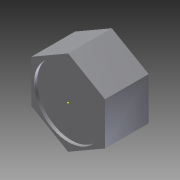
# Autodesk Inventor part: Поз10 Заглушка
Saved by Autodesk Inventor 2012 SP2 (Build 160219200, 219)
## iProperties
Created: 2014-04-06
Part Number: Поз10 Заглушка
Material: Default
Document SubType Name: Modeling
Designer: N750
Density: 1 g/cm^3
Author: N750
Autodesk Inventor part; units mm, degrees
ref_plane "YZ Plane" through (0, 0, 0) normal (1, 0, 0) x (0, 1, 0)
ref_plane "XZ Plane" through (0, 0, 0) normal (0, 1, 0) x (-1, 0, 0)
ref_plane "XY Plane" through (0, 0, 0) normal (0, 0, 1) x (1, 0, 0)
sketch "Эскиз1" plane through (0, 0, 0) normal (0, 0, 1) x (1, 0, 0)
  point P0 (0, 0)
sketch "Эскиз2" plane through (0, 0, 0) normal (0, 1, 0) x (-1, 0, 0)
  line L0 (0, 15.5885) -> (13.5, 7.7942)
  line L1 (13.5, 7.7942) -> (13.5, -7.7942)
  line L2 (13.5, -7.7942) -> (0, -15.5885)
  line L3 (0, -15.5885) -> (-13.5, -7.7942)
  line L4 (-13.5, -7.7942) -> (-13.5, 7.7942)
  line L5 (-13.5, 7.7942) -> (0, 15.5885)
  point P0 (0, 0)
  point P1 (0, 0)
  dimension "d0" = 27
  constraints: 12 end point, 1 coincident, 13 other
  measures "d0" distance of L1.end L3.end
extrude "Выдавливание1" add sketch "Эскиз2" along normal blind 16
sketch "Эскиз3" plane through (0, 0, 0) normal (0, -1, 0) x (1, 0, 0)
  circle A0 centre (0, 0) radius 12.5
  dimension "d3" = 25
  constraints: 1 centre point, 1 coincident
  measures "d3" diameter of A0
sketch "Эскиз4" plane through (0, 16, 0) normal (0, 1, 0) x (1, 0, 0)
  circle A0 centre (0, 0) radius 10.2935
  dimension "d4" = 20.587
  constraints: 1 centre point, 1 coincident
  measures "d4" diameter of A0
extrude "Выдавливание2" cut sketch "Эскиз4" against normal blind 12
thread "Резьба1" size "G 5/8-14" standard "BSP Pipe Threads" length 10 offset 2
chamfer "Фаска1" distance 1.6 angle 45 1 edges at (-10.2935, 16, 0) measured on face at (10.1602, 8, 1.6512)
extrude "Выдавливание3" cut sketch "Эскиз3" against normal blind 1.154
